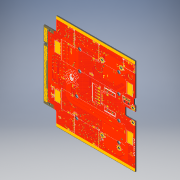
# Autodesk Inventor part: EPS_PCB
Saved by Autodesk Inventor 2018 (Build 220112000, 112)
## iProperties
Created: 2018-01-15
Part Number: EPS_PCB
Material: Epoxy Resin
Document SubType Name: Modeling
Designer: Bradley
Density: 1.14 g/cm^3
Appearance: Smooth - Dark Gray
Author: Bradley
Revision Number: 3
Autodesk Inventor part; units mm, degrees
ref_plane "YZ Plane" through (0, 0, 0) normal (1, 0, 0) x (0, 1, 0)
ref_plane "XZ Plane" through (0, 0, 0) normal (0, 1, 0) x (-1, 0, 0)
ref_plane "XY Plane" through (0, 0, 0) normal (0, 0, 1) x (1, 0, 0)
sketch "Sketch1" plane through (0, 0, 0) normal (0, 0, 1) x (1, 0, 0)
  line L0 (0, 33.8) -> (12.5, 33.8)
  line L1 (12.5, 33.8) -> (12.5, 47.9)
  line L2 (12.5, 47.9) -> (91.4, 47.9)
  line L3 (91.4, 47.9) -> (91.4, -47.9)
  line L4 (91.4, -47.9) -> (12.5, -47.9)
  line L5 (12.5, -47.9) -> (12.5, -33.8)
  line L6 (12.5, -33.8) -> (0, -33.8)
  line L7 (0, -33.8) -> (0, 33.8)
  line L8 (-4.5, 48) -> (91.5, 48) construction
  line L9 (91.5, 48) -> (91.5, -48) construction
  line L10 (91.5, -48) -> (-4.5, -48) construction
  line L11 (-4.5, -48) -> (-4.5, 48) construction
  line L12 (-4.4, 47.9) -> (-3.4, 47.9) construction
  line L13 (-3.4, 47.9) -> (-3.4, -47.9) construction
  line L14 (-3.4, -47.9) -> (-4.4, -47.9) construction
  line L15 (-4.4, -47.9) -> (-4.4, 47.9) construction
  point P0 (0, 0)
  point P1 (0, 0)
  point P2 (-4.5, 0)
  dimension "d0" = 67.6
  dimension "d1" = 95.8
  dimension "d2" = 91.4
  dimension "d3" = 12.5
  dimension "d20" = 96
  dimension "d21" = 96
  dimension "d22" = 0.1
  dimension "d23" = 0.1
  dimension "d24" = 1
  dimension "d25" = 0.1
  dimension "d26" = 3.4
  constraints: 32 end point, 8 perpendicular, 4 parallel, 3 collinear, 3 horizontal, 2 midpoint, 2 point on line, 1 coincident, 1 horizontal alignment
  measures "d0" distance of L6.end L0.start
  measures "d1" distance of L2.end L3.end
  measures "d2" distance between parallel lines of L7 L3
  measures "d3" distance of L0.start L0.end
  measures "d20" distance of L8.start L8.end
  measures "d21" distance of L10.end L8.start
  measures "d22" distance between parallel lines of L2 L8
  measures "d23" distance between parallel lines of L9 L3
  measures "d24" distance between parallel lines of L15 L13
  measures "d25" distance between parallel lines of L15 L11
  measures "d26" distance between parallel lines of L7 L13
extrude "Extrusion1" add sketch "Sketch1" along normal mid plane 1
sketch "Sketch3" plane through (0, 0, 0.5) normal (0, 0, 1) x (1, 0, 0)
  circle A0 centre (6, 31.8) radius 0.9
  circle A1 centre (6, -31.8) radius 0.9
  point P0 (0, 0)
  dimension "d9" = 1.8
  dimension "d10" = 6
  dimension "d11" = 31.8
  dimension "d12" = 31.8
  constraints: 2 centre point, 1 equal radius, 1 vertical alignment
  measures "d9" diameter of A0
  measures "d10" horizontal distance of point (0, 0) A0.centre
  measures "d11" vertical distance of point (0, 0) A0.centre
  measures "d12" vertical distance of A1.centre point (0, 0)
extrude "Extrusion3" cut sketch "Sketch3" against normal through all
sketch "Sketch4" plane through (0, 0, 0.5) normal (0, 0, 1) x (1, 0, 0)
  circle A0 centre (6, 31.8) radius 0.9 projected
  circle A1 centre (6, -31.8) radius 0.9 projected
  line L0 (91.4, -47.9) -> (91.4, 47.9) projected
  line L1 (12.5, 47.9) -> (12.5, 33.8) projected
  line L2 (12.5, 33.8) -> (0, 33.8) projected
  line L3 (0, 33.8) -> (0, -33.8) projected
  line L4 (0, -33.8) -> (12.5, -33.8) projected
  line L5 (12.5, -33.8) -> (12.5, -47.9) projected
  line L6 (0, 18.95) -> (3.5, 18.95)
  arc A2 (3.5, 17.95) -> (3.5, 18.95) centre (3.5, 18.45) ccw
  line L7 (3.5, 17.95) -> (0, 17.95)
  line L8 (12.5, -47.9) -> (91.4, -47.9) projected
  line L9 (91.4, 47.9) -> (12.5, 47.9) projected
  point P0 (0, 0)
  dimension "d15" = 17.95
  dimension "d16" = 3.5
  dimension "d17" = 1
  constraints: 4 end point, 2 point on circle, 2 point on line, 2 tangent, 1 centre point, 1 horizontal, 1 perpendicular
  measures "d15" distance from line of point (0, 0) L7
  measures "d16" distance from line of A2.centre L3
  measures "d17" distance between parallel lines of L7 L6
extrude "Extrusion4" cut sketch "Sketch4" against normal through all contours L3 L6 A2 L7
sketch "Sketch5" plane through (0, 0, 0.5) normal (0, 0, 1) x (1, 0, 0)
  line L0 (89.1, 6.3) -> (89.1, -6.3) construction
  line L1 (91.4, -47.9) -> (91.4, 47.9) projected
  line L2 (0, 17.95) -> (0, -33.8) projected
  point P0 (0, 0)
  point P1 (89.1, 0)
  point P2 (91.4, 0)
  point P3 (91.4, -45.4)
  point P4 (91.4, 45.4)
  dimension "d29" = 12.6
  dimension "d69" = 89.1
  constraints: 2 coincident, 2 end point, 2 midpoint, 1 horizontal alignment, 1 vertical
  measures "d29" distance of L0.start L0.end
  measures "d69" distance between parallel lines of L0 L2
hole "Hole1" at (89.1, 6.3, 0.5) at (89.1, -6.3, 0.5) direction (0, 0, -1) diameter 2.2 end through all clearance for "Socket Head Cap Screw" size "M2" standard "Ansi Metric M Profile"
sketch "Sketch6" plane through (0, 0, 0.5) normal (0, 0, 1) x (1, 0, 0)
  circle A0 centre (89.1, 6.3) radius 1.1 projected
  circle A1 centre (89.1, -6.3) radius 1.1 projected
  line L0 (0, 18.95) -> (3.5, 18.95) projected
  arc A2 (3.5, 17.95) -> (3.5, 18.95) centre (3.5, 18.45) ccw projected
  line L1 (3.5, 17.95) -> (0, 17.95) projected
  line L2 (0, 17.95) -> (0, -33.8) projected
  line L3 (0, -33.8) -> (12.5, -33.8) projected
  line L4 (12.5, -33.8) -> (12.5, -47.9) projected
  line L5 (91.4, -47.9) -> (91.4, 47.9) projected
  line L6 (12.5, 47.9) -> (12.5, 33.8) projected
  line L7 (12.5, 33.8) -> (0, 33.8) projected
  line L8 (0, 33.8) -> (0, 18.95) projected
  circle A3 centre (6, -31.8) radius 0.9 projected
  circle A4 centre (6, 31.8) radius 0.9 projected
  line L9 (91.4, 45.4) -> (91.4, -45.4) projected
  line L10 (91.4, 4) -> (82.4, 4)
  arc A5 (82.4, 4) -> (81.4, 3) centre (82.4, 3) ccw
  line L11 (81.4, 3) -> (81.4, -3)
  arc A6 (81.4, -3) -> (82.4, -4) centre (82.4, -3) ccw
  line L12 (82.4, -4) -> (91.4, -4)
  circle A7 centre (90.7, 13.2) radius 0.7 construction
  circle A8 centre (90.7, 11.8) radius 0.7 construction
  line L13 (91.4, 15.5) -> (90.9, 15.5)
  arc A9 (90.9, 15.5) -> (89.9, 14.5) centre (90.9, 14.5) ccw
  line L14 (89.9, 14.5) -> (89.9, 10.5)
  arc A10 (89.9, 10.5) -> (90.9, 9.5) centre (90.9, 10.5) ccw
  line L15 (90.9, 9.5) -> (91.4, 9.5)
  line L16 (91.4, -45.4) -> (91.4, 45.4) construction
  line L17 (89.9, 12.5) -> (91.4, 12.5) construction
  line L18 (12.5, -47.9) -> (91.4, -47.9) projected
  line L19 (91.4, 47.9) -> (12.5, 47.9) projected
  point P0 (0, 0)
  point P1 (81.4, 0)
  dimension "d37" = 1
  dimension "d38" = 8
  dimension "d39" = 1.2
  dimension "d40" = 10
  dimension "d65" = 1.4
  dimension "d66" = 1.5
  dimension "d67" = 6
  dimension "d68" = 12.5
  dimension "d70" = 9.5
  dimension "d71" = 15.5
  constraints: 14 end point, 12 tangent, 8 point on circle, 7 perpendicular, 6 centre point, 5 point on line, 3 equal radius, 2 midpoint, 1 horizontal alignment, 1 parallel
  measures "d37" radius of A5
  measures "d38" distance between parallel lines of L12 L10
  measures "d39" distance edge to line of A0 L10
  measures "d40" distance between parallel lines of L5 L11
  measures "d65" diameter of A7
  measures "d66" distance between parallel lines of L5 L14
  measures "d67" distance between parallel lines of L15 L13
  measures "d68" distance from line of point (0, 0) L17
  measures "d70" distance from line of L15 point (0, 0)
  measures "d71" distance from line of point (0, 0) L13
extrude "Extrusion5" cut sketch "Sketch6" against normal through all contours L5 L15 A10 L14 A9 L13 | L5 L12 A6 L11 A5 L10
sketch "Sketch7" plane through (0, 0, 0.5) normal (0, 0, 1) x (1, 0, 0)
  line L0 (80.65, 7.93) -> (84.65, 7.93) construction
  line L1 (91.4, 4) -> (91.4, 9.5) projected
  point P0 (0, 0)
  point P1 (91.4, 45.4)
  dimension "d43" = 7.93
  dimension "d44" = 6.75
  dimension "d45" = 4
  constraints: 2 coincident, 2 end point, 1 horizontal
  measures "d43" distance from line of point (0, 0) L0
  measures "d44" distance from line of L1 L0.end
  measures "d45" distance of L0.start L0.end
hole "Hole2" at (80.65, 7.93, 0.5) at (84.65, 7.93, 0.5) direction (0, 0, -1) diameter 1.7 end through all
fillet "Fillet1" radius 0.5 12 edges at (91.4, 4, 0) (91.4, -4, 0) (91.4, 9.5, 0) (91.4, 15.5, 0) (91.4, 47.9, 0) (12.5, 47.9, 0) (0, 33.8, 0) (0, 18.95, 0) (0, 17.95, 0) (0, -33.8, 0) (12.5, -47.9, 0) (91.4, -47.9, 0)
fillet "Fillet1" radius 1 2 edges at (12.5, 33.8, 0) (12.5, -33.8, 0)
sketch "Sketch8" plane through (0, 0, 0.5) normal (0, 0, 1) x (1, 0, 0)
  arc A0 (91.4, -4.5) -> (90.9, -4) centre (90.9, -4.5) ccw projected
  line L0 (90.9, -4) -> (82.4, -4) projected
  arc A1 (81.4, -3) -> (82.4, -4) centre (82.4, -3) ccw projected
  line L1 (81.4, -3) -> (81.4, 3) projected
  arc A2 (82.4, 4) -> (81.4, 3) centre (82.4, 3) ccw projected
  line L2 (82.4, 4) -> (90.9, 4) projected
  arc A3 (90.9, 4) -> (91.4, 4.5) centre (90.9, 4.5) ccw projected
  line L3 (91.4, 4.5) -> (91.4, 9) projected
  line L4 (12.5, 47.4) -> (12.5, 34.8) projected
  arc A4 (11.5, 33.8) -> (12.5, 34.8) centre (11.5, 34.8) ccw projected
  line L5 (11.5, 33.8) -> (0.5, 33.8) projected
  line L6 (0, 17.45) -> (0, -33.3) projected
  line L7 (0.5, 18.95) -> (3.5, 18.95) projected
  arc A5 (3.5, 17.95) -> (3.5, 18.95) centre (3.5, 18.45) ccw projected
  line L8 (3.5, 17.95) -> (0.5, 17.95) projected
  line L9 (0, 33.3) -> (0, 19.45) projected
  line L10 (0.5, -33.8) -> (11.5, -33.8) projected
  arc A6 (12.5, -34.8) -> (11.5, -33.8) centre (11.5, -34.8) ccw projected
  line L11 (12.5, -34.8) -> (12.5, -47.4) projected
  line L12 (91.4, 16) -> (91.4, 47.4) projected
  circle A7 centre (80.65, 7.93) radius 0.85 projected
  circle A8 centre (84.65, 7.93) radius 0.85 projected
  circle A9 centre (6, 31.8) radius 0.9 projected
  circle A10 centre (6, -31.8) radius 0.9 projected
  circle A11 centre (89.1, -6.3) radius 1.1 projected
  circle A12 centre (89.1, 6.3) radius 1.1 projected
  line L13 (75, 30.5) -> (75, 11.5) construction
  line L14 (33, -11.5) -> (33, -30.5) construction
  line L15 (75, -11.5) -> (75, -30.5) construction
  line L16 (0, 0) -> (81.4, 0) construction
  arc A13 (89.9, 10.5) -> (90.9, 9.5) centre (90.9, 10.5) ccw projected
  line L17 (89.9, 10.5) -> (89.9, 14.5) projected
  arc A14 (90.9, 15.5) -> (89.9, 14.5) centre (90.9, 14.5) ccw projected
  line L18 (91.4, -47.4) -> (91.4, -4.5) projected
  arc A15 (90.9, 15.5) -> (91.4, 16) centre (90.9, 16) ccw projected
  arc A16 (91.4, 9) -> (90.9, 9.5) centre (90.9, 9) ccw projected
  arc A17 (90.9, -47.9) -> (91.4, -47.4) centre (90.9, -47.4) ccw projected
  arc A18 (91.4, 47.4) -> (90.9, 47.9) centre (90.9, 47.4) ccw projected
  line L19 (90.9, 47.9) -> (13, 47.9) projected
  arc A19 (13, 47.9) -> (12.5, 47.4) centre (13, 47.4) ccw projected
  arc A20 (0.5, 33.8) -> (0, 33.3) centre (0.5, 33.3) ccw projected
  arc A21 (0, 19.45) -> (0.5, 18.95) centre (0.5, 19.45) ccw projected
  arc A22 (0.5, 17.95) -> (0, 17.45) centre (0.5, 17.45) ccw projected
  arc A23 (0, -33.3) -> (0.5, -33.8) centre (0.5, -33.3) ccw projected
  arc A24 (12.5, -47.4) -> (13, -47.9) centre (13, -47.4) ccw projected
  line L20 (13, -47.9) -> (90.9, -47.9) projected
  line L21 (36, 30.5) -> (36, 11.5) construction
  point P0 (75, 21)
  point P1 (75, -21)
  point P2 (33, -21)
  dimension "d54" = 21
  dimension "d55" = 33
  dimension "d56" = 75
  dimension "d57" = 19
  dimension "d73" = 36
  constraints: 10 end point, 6 coincident, 4 midpoint, 4 vertical, 3 horizontal alignment, 2 symmetric about line, 1 parallel
  measures "d54" vertical distance of point (33, -21) L16.start
  measures "d55" distance between parallel lines of L14 L9
  measures "d56" distance between parallel lines of L15 L9
  measures "d57" distance of L14.start L14.end
  measures "d73" distance between parallel lines of L9 L21
hole "Hole3" at (36, 30.5, 0.5) at (36, 11.5, 0.5) at (75, 11.5, 0.5) at (75, 30.5, 0.5) at (75, -11.5, 0.5) at (75, -30.5, 0.5) at (33, -30.5, 0.5) at (33, -11.5, 0.5) direction (0, 0, -1) diameter 3 end through all
sketch "Sketch10" plane through (0, 0, 0.5) normal (0, 0, 1) x (1, 0, 0)
  line L0 (0, 33.3) -> (0, 19.45) projected
  point P0 (0, 0)
  point P1 (58.3, 32.5)
  point P2 (77.3, 35)
  point P3 (58.4, -32.5)
  point P4 (75.1, -35)
  dimension "d74" = 58.3
  dimension "d75" = 32.5
  dimension "d76" = 35
  dimension "d77" = 77.3
  dimension "d78" = 75.1
  dimension "d79" = 35
  dimension "d80" = 32.5
  dimension "d81" = 58.4
  measures "d74" distance from line of point (58.3, 32.5) L0
  measures "d75" vertical distance of point (0, 0) point (58.3, 32.5)
  measures "d76" vertical distance of point (0, 0) point (77.3, 35)
  measures "d77" horizontal distance of point (77.3, 35) point (0, 0)
  measures "d78" horizontal distance of point (75.1, -35) point (0, 0)
  measures "d79" vertical distance of point (0, 0) point (75.1, -35)
  measures "d80" vertical distance of point (0, 0) point (58.4, -32.5)
  measures "d81" horizontal distance of point (58.4, -32.5) point (0, 0)
hole "Hole4" at (58.3, 32.5, 0.5) at (77.3, 35, 0.5) at (58.4, -32.5, 0.5) at (75.1, -35, 0.5) direction (0, 0, -1) diameter 2.2 end through all
sketch "Sketch11" plane through (0, 0, 0.5) normal (0, 0, 1) x (1, 0, 0)
  line L0 (0, 47.8798) -> (91.4, 47.8798) construction
  line L1 (91.4, 47.8798) -> (91.4, -47.8798) construction
  line L2 (91.4, -47.8798) -> (0, -47.8798) construction
  line L3 (0, -47.8798) -> (0, 47.8798) construction
  circle A0 centre (58.4, -32.5) radius 1.1 projected
  circle A1 centre (58.3, 32.5) radius 1.1 projected
  circle A2 centre (77.3, 35) radius 1.1 projected
  circle A3 centre (75.1, -35) radius 1.1 projected
  circle A4 centre (33, -30.5) radius 1.5 projected
  circle A5 centre (75, -11.5) radius 1.5 projected
  circle A6 centre (75, 11.5) radius 1.5 projected
  circle A7 centre (36, 30.5) radius 1.5 projected
  circle A8 centre (36, 11.5) radius 1.5 projected
  circle A9 centre (75, 30.5) radius 1.5 projected
  circle A10 centre (75, -30.5) radius 1.5 projected
  circle A11 centre (33, -11.5) radius 1.5 projected
  arc A12 (90.9, -47.9) -> (91.4, -47.4) centre (90.9, -47.4) ccw projected
  line L4 (91.4, -47.4) -> (91.4, -4.5) projected
  arc A13 (91.4, -4.5) -> (90.9, -4) centre (90.9, -4.5) ccw projected
  line L5 (90.9, -4) -> (82.4, -4) projected
  arc A14 (81.4, -3) -> (82.4, -4) centre (82.4, -3) ccw projected
  line L6 (81.4, -3) -> (81.4, 3) projected
  arc A15 (82.4, 4) -> (81.4, 3) centre (82.4, 3) ccw projected
  line L7 (82.4, 4) -> (90.9, 4) projected
  arc A16 (90.9, 4) -> (91.4, 4.5) centre (90.9, 4.5) ccw projected
  line L8 (91.4, 4.5) -> (91.4, 9) projected
  arc A17 (91.4, 9) -> (90.9, 9.5) centre (90.9, 9) ccw projected
  arc A18 (89.9, 10.5) -> (90.9, 9.5) centre (90.9, 10.5) ccw projected
  line L9 (89.9, 10.5) -> (89.9, 14.5) projected
  arc A19 (90.9, 15.5) -> (89.9, 14.5) centre (90.9, 14.5) ccw projected
  arc A20 (90.9, 15.5) -> (91.4, 16) centre (90.9, 16) ccw projected
  line L10 (91.4, 16) -> (91.4, 47.4) projected
  arc A21 (91.4, 47.4) -> (90.9, 47.9) centre (90.9, 47.4) ccw projected
  line L11 (90.9, 47.9) -> (13, 47.9) projected
  arc A22 (13, 47.9) -> (12.5, 47.4) centre (13, 47.4) ccw projected
  line L12 (12.5, 47.4) -> (12.5, 34.8) projected
  arc A23 (11.5, 33.8) -> (12.5, 34.8) centre (11.5, 34.8) ccw projected
  line L13 (11.5, 33.8) -> (0.5, 33.8) projected
  arc A24 (0.5, 33.8) -> (0, 33.3) centre (0.5, 33.3) ccw projected
  line L14 (0, 33.3) -> (0, 19.45) projected
  arc A25 (0, 19.45) -> (0.5, 18.95) centre (0.5, 19.45) ccw projected
  line L15 (0.5, 18.95) -> (3.5, 18.95) projected
  arc A26 (3.5, 17.95) -> (3.5, 18.95) centre (3.5, 18.45) ccw projected
  line L16 (3.5, 17.95) -> (0.5, 17.95) projected
  arc A27 (0.5, 17.95) -> (0, 17.45) centre (0.5, 17.45) ccw projected
  line L17 (0, 17.45) -> (0, -33.3) projected
  arc A28 (0, -33.3) -> (0.5, -33.8) centre (0.5, -33.3) ccw projected
  line L18 (0.5, -33.8) -> (11.5, -33.8) projected
  arc A29 (12.5, -34.8) -> (11.5, -33.8) centre (11.5, -34.8) ccw projected
  line L19 (12.5, -34.8) -> (12.5, -47.4) projected
  arc A30 (12.5, -47.4) -> (13, -47.9) centre (13, -47.4) ccw projected
  line L20 (13, -47.9) -> (90.9, -47.9) projected
  circle A31 centre (89.1, 6.3) radius 1.1 projected
  circle A32 centre (89.1, -6.3) radius 1.1 projected
  circle A33 centre (6, -31.8) radius 0.9 projected
  circle A34 centre (6, 31.8) radius 0.9 projected
  circle A35 centre (84.65, 7.93) radius 0.85 projected
  circle A36 centre (80.65, 7.93) radius 0.85 projected
  line L21 (0, 17.45) -> (0, -33.3) projected
  line L22 (91.4, 16) -> (91.4, 47.4) projected
  point P0 (0, 0)
  constraints: 2 collinear, 1 midpoint, 2 other
decal "Decal1"
sketch "Sketch12" plane through (0, 0, -0.5) normal (0, 0, -1) x (-1, 0, 0)
  circle A0 centre (-58.4, -32.5) radius 1.1 projected
  circle A1 centre (-58.3, 32.5) radius 1.1 projected
  circle A2 centre (-77.3, 35) radius 1.1 projected
  circle A3 centre (-75.1, -35) radius 1.1 projected
  circle A4 centre (-33, -30.5) radius 1.5 projected
  circle A5 centre (-75, -11.5) radius 1.5 projected
  circle A6 centre (-75, 11.5) radius 1.5 projected
  circle A7 centre (-36, 30.5) radius 1.5 projected
  circle A8 centre (-36, 11.5) radius 1.5 projected
  circle A9 centre (-75, 30.5) radius 1.5 projected
  circle A10 centre (-75, -30.5) radius 1.5 projected
  circle A11 centre (-33, -11.5) radius 1.5 projected
  circle A12 centre (-6, -31.8) radius 0.9 projected
  circle A13 centre (-6, 31.8) radius 0.9 projected
  circle A14 centre (-89.1, -6.3) radius 1.1 projected
  circle A15 centre (-89.1, 6.3) radius 1.1 projected
  circle A16 centre (-84.65, 7.93) radius 0.85 projected
  circle A17 centre (-80.65, 7.93) radius 0.85 projected
  arc A18 (-91.4, -47.4) -> (-90.9, -47.9) centre (-90.9, -47.4) ccw projected
  line L0 (-90.9, -47.9) -> (-13, -47.9) projected
  arc A19 (-13, -47.9) -> (-12.5, -47.4) centre (-13, -47.4) ccw projected
  line L1 (-12.5, -47.4) -> (-12.5, -34.8) projected
  arc A20 (-11.5, -33.8) -> (-12.5, -34.8) centre (-11.5, -34.8) ccw projected
  line L2 (-11.5, -33.8) -> (-0.5, -33.8) projected
  arc A21 (-0.5, -33.8) -> (0, -33.3) centre (-0.5, -33.3) ccw projected
  line L3 (0, -33.3) -> (0, 17.45) projected
  arc A22 (0, 17.45) -> (-0.5, 17.95) centre (-0.5, 17.45) ccw projected
  line L4 (-0.5, 17.95) -> (-3.5, 17.95) projected
  arc A23 (-3.5, 18.95) -> (-3.5, 17.95) centre (-3.5, 18.45) ccw projected
  line L5 (-3.5, 18.95) -> (-0.5, 18.95) projected
  arc A24 (-0.5, 18.95) -> (0, 19.45) centre (-0.5, 19.45) ccw projected
  line L6 (0, 19.45) -> (0, 33.3) projected
  arc A25 (0, 33.3) -> (-0.5, 33.8) centre (-0.5, 33.3) ccw projected
  line L7 (-0.5, 33.8) -> (-11.5, 33.8) projected
  arc A26 (-12.5, 34.8) -> (-11.5, 33.8) centre (-11.5, 34.8) ccw projected
  line L8 (-12.5, 34.8) -> (-12.5, 47.4) projected
  arc A27 (-12.5, 47.4) -> (-13, 47.9) centre (-13, 47.4) ccw projected
  line L9 (-13, 47.9) -> (-90.9, 47.9) projected
  arc A28 (-90.9, 47.9) -> (-91.4, 47.4) centre (-90.9, 47.4) ccw projected
  line L10 (-91.4, 47.4) -> (-91.4, 16) projected
  arc A29 (-91.4, 16) -> (-90.9, 15.5) centre (-90.9, 16) ccw projected
  arc A30 (-89.9, 14.5) -> (-90.9, 15.5) centre (-90.9, 14.5) ccw projected
  line L11 (-89.9, 14.5) -> (-89.9, 10.5) projected
  arc A31 (-90.9, 9.5) -> (-89.9, 10.5) centre (-90.9, 10.5) ccw projected
  arc A32 (-90.9, 9.5) -> (-91.4, 9) centre (-90.9, 9) ccw projected
  line L12 (-91.4, 9) -> (-91.4, 4.5) projected
  arc A33 (-91.4, 4.5) -> (-90.9, 4) centre (-90.9, 4.5) ccw projected
  line L13 (-90.9, 4) -> (-82.4, 4) projected
  arc A34 (-81.4, 3) -> (-82.4, 4) centre (-82.4, 3) ccw projected
  line L14 (-81.4, 3) -> (-81.4, -3) projected
  arc A35 (-82.4, -4) -> (-81.4, -3) centre (-82.4, -3) ccw projected
  line L15 (-82.4, -4) -> (-90.9, -4) projected
  arc A36 (-90.9, -4) -> (-91.4, -4.5) centre (-90.9, -4.5) ccw projected
  line L16 (-91.4, -4.5) -> (-91.4, -47.4) projected
  line L17 (0, -33.3) -> (0, 17.45) projected
  line L18 (-91.4, 47.8917) -> (0, 47.8917) construction
  line L19 (0, 47.8917) -> (0, -47.8917) construction
  line L20 (0, -47.8917) -> (-91.4, -47.8917) construction
  line L21 (-91.4, -47.8917) -> (-91.4, 47.8917) construction
  line L22 (-91.4, 47.4) -> (-91.4, 16) projected
  point P0 (0, 0)
  constraints: 2 collinear, 1 midpoint, 2 other
decal "Decal2"
sketch "Sketch13" plane through (0, 0, 0.5) normal (0, 0, 1) x (1, 0, 0)
  point P0 (0, 0)
  point P1 (89.96, 41.605)
  point P2 (61.8, 38.5)
  point P3 (62.4, 38.5)
  point P4 (62.4, 39.1)
  point P5 (63, 39.1)
  point P6 (63, 39.7)
  point P7 (40.8, 35.695)
  point P8 (61.1, 39.8)
  point P9 (60.5, 39.8)
  point P10 (60.5, 39.2)
  point P11 (59.9, 39.2)
  point P12 (59.9, 38.6)
  point P13 (34.6, 34.5)
  point P14 (33.21, -3.955)
  point P15 (35.14, -4.665)
  point P16 (38, -33.2)
  point P17 (42.6, -39.6)
  point P18 (40.095, -41.49)
  point P19 (54.71, -30.72)
  point P20 (50, -39.6)
  point P21 (47.5, -41.7)
  point P22 (29.8, 43.6)
  point P23 (51, 41.7)
  point P24 (40.6, 40.96)
  point P25 (43.1, 43.1)
  point P26 (58.4, -6.46)
  point P27 (76.84, -5.14)
  point P28 (77.5, 5.4)
  point P29 (55.26, -42.83)
  point P30 (27.48, -21.06)
  point P31 (36.425, -25.76)
  point P32 (88.9, 21.15)
  point P33 (89.45, 20.8)
  point P34 (88.9, 20.45)
  point P35 (89.45, 20.1)
  point P36 (88.9, 19.75)
  point P37 (89.45, 19.4)
  point P38 (88.9, 19.05)
  point P39 (79.82, -3.995)
  point P40 (85.12, 31.545)
  point P41 (52.8, 22)
  point P42 (51.16, 44.12)
  point P43 (36.315, 43.16)
  point P44 (34, 40.7)
  point P45 (29.26, -22.34)
  point P46 (56.36, -42.83)
  point P47 (86.1, -15.5)
  point P48 (86.8, -15.5)
  point P49 (87.5, -15.5)
  point P50 (88.2, -15.5)
  point P51 (88.9, -15.7)
  point P52 (89, -16.4)
  point P53 (89, -17.1)
  point P54 (89, -17.8)
  point P55 (89, -18.5)
  point P56 (36.38, -26.57)
  point P57 (78.1, -7)
  point P58 (79.355, -3.255)
  point P59 (51.1, 42.9)
  point P60 (10.2, -23.5)
  point P61 (7.6, -20.8)
  point P62 (10.4, -20.8)
  point P63 (11, -23.5)
  point P64 (10.2, -16.8)
  point P65 (7.6, -14.1)
  point P66 (11, -16.8)
  point P67 (10.85, -14.23)
  point P68 (16.5, -14.5)
  point P69 (16.5, -15.3)
  point P70 (17.1, -15.7)
  point P71 (17.1, -14.9)
  point P72 (17.1, -14.1)
  point P73 (26.79, -20.74)
  point P74 (53.3, -24.9)
  point P75 (65.155, 10.12)
  point P76 (52, 22.1)
  point P77 (20, 6.69)
  point P78 (20, 3.69)
  point P79 (20, 0.69)
  point P80 (24.54, 7.29)
  point P81 (24.1, 5.25)
  point P82 (24.1, 2.15)
  point P83 (24.125, -0.96)
  point P84 (78.3, -37.4)
  point P85 (81.2, -17.1)
  point P86 (81.2, -17.9)
  point P87 (81.2, -18.7)
  point P88 (81.2, -19.5)
  point P89 (80.6, -19.1)
  point P90 (80.6, -18.3)
  point P91 (80.6, -17.5)
  point P92 (79.5, -38.9)
  point P93 (60.7, -41.8)
  point P94 (54.9, -25.4)
  point P95 (49.9, -17.2)
  point P96 (78, -17)
  point P97 (77.2, -17)
  point P98 (75.3, 8)
  point P99 (75.7, 7.5)
  point P100 (74.9, 7.5)
  point P101 (86.23, 30.36)
  point P102 (87, 30.2)
  point P103 (16.5, 5.53)
  point P104 (16.5, 2.53)
  point P105 (16.5, -0.47)
  point P106 (21.1, 6.97)
  point P107 (21.1, 3.97)
  point P108 (21.1, 0.97)
  point P109 (21.1, -2.03)
  point P110 (17.6, -2.4)
  point P111 (18.4, -2.4)
  point P112 (19.2, -2.4)
  point P113 (20, -2.4)
  point P114 (20.4, -3.1)
  point P115 (19.6, -3.1)
  point P116 (18.8, -3.1)
  point P117 (18, -3.1)
  point P118 (28.5, -3.2)
  point P119 (28.5, -4)
  point P120 (28.5, -4.8)
  point P121 (28.5, -5.6)
  point P122 (29.1, -5.2)
  point P123 (29.1, -4.4)
  point P124 (29.1, -3.6)
  point P125 (27.6, 22.4)
  point P126 (27.6, 23)
  point P127 (27.6, 23.7)
  point P128 (27.6, 24.3)
  point P129 (27.05, 24)
  point P130 (27.1, 23.35)
  point P131 (28.5, -11.42)
  point P132 (32.13, -21.7)
  point P133 (21.2, -42.1)
  point P134 (29.295, -43.15)
  point P135 (34.66, -26.63)
  point P136 (54.85, -20.36)
  point P137 (56.64, -20.36)
  point P138 (73, 41.8)
  point P139 (84.36, 31.55)
  point P140 (53.67, 21.255)
  point P141 (58.1, 22.8)
  point P142 (19.26, -22.78)
  point P143 (43.945, -10.34)
  point P144 (79.28, 4.89)
  point P145 (79.375, 14.54)
  point P146 (83.96, 26.46)
  point P147 (43.4, -40.4)
  point P148 (52.1, -33.5)
  point P149 (40.1, -40.6)
  point P150 (49.4, -33.9)
  point P151 (50.7, -40.5)
  point P152 (52.6, -38)
  point P153 (47.64, -39.63)
  point P154 (51.6, -36.4)
  point P155 (35.23, 40.2)
  point P156 (35.395, 38.8)
  point P157 (37.02, 41.69)
  point P158 (36.155, 38.8)
  point P159 (40.545, 42.945)
  point P160 (37.685, 38.8)
  point P161 (43.645, 41.71)
  point P162 (40.18, 38.76)
  point P163 (60.01, -1.17)
  point P164 (77, -3.8)
  point P165 (64.23, -0.73)
  point P166 (59.32, -1.49)
  point P167 (77.56, -5.495)
  point P168 (64.255, -1.49)
  point P169 (28.24, -21.06)
  point P170 (53.1, -25.7)
  point P171 (26.13, -20.36)
  point P172 (54.1, -24.7)
  point P173 (15.8, 40.45)
  point P174 (22.3, 38.45)
  point P175 (15.3, -4.2)
  point P176 (17, -5.2)
  point P177 (13.71, -10.51)
  point P178 (29.895, -6.39)
  point P179 (25.4, 40.45)
  point P180 (31.6, 38)
  point P181 (31.12, 30.22)
  point P182 (28.48, -10.66)
  point P183 (19.6, -13.6)
  point P184 (28.9, -38.5)
  point P185 (27.58, -34.4)
  point P186 (47.6, -27.75)
  point P187 (44.2, -21.8)
  point P188 (37.24, -26.61)
  point P189 (35.26, -35.79)
  point P190 (57.925, 25.16)
  point P191 (51.6, 27.8)
  point P192 (51.6, 25.9)
  point P193 (47.97, 26.905)
  point P194 (43.625, 31.08)
  point P195 (71.1, -41.92)
  point P196 (55.7, -25.6)
  point P197 (20, 27.59)
  point P198 (21.9, 30.59)
  point P199 (20, 24.59)
  constraints: 629 other
hole "Hole5" at (89.96, 41.605, 0.5) at (61.8, 38.5, 0.5) at (62.4, 38.5, 0.5) at (62.4, 39.1, 0.5) at (63, 39.1, 0.5) at (63, 39.7, 0.5) at (40.8, 35.695, 0.5) at (61.1, 39.8, 0.5) at (60.5, 39.8, 0.5) at (60.5, 39.2, 0.5) at (59.9, 39.2, 0.5) at (59.9, 38.6, 0.5) at (34.6, 34.5, 0.5) at (33.21, -3.955, 0.5) at (35.14, -4.665, 0.5) at (38, -33.2, 0.5) at (42.6, -39.6, 0.5) at (40.095, -41.49, 0.5) at (54.71, -30.72, 0.5) at (50, -39.6, 0.5) at (47.5, -41.7, 0.5) at (29.8, 43.6, 0.5) at (51, 41.7, 0.5) at (40.6, 40.96, 0.5) at (43.1, 43.1, 0.5) at (58.4, -6.46, 0.5) at (76.84, -5.14, 0.5) at (77.5, 5.4, 0.5) at (55.26, -42.83, 0.5) at (27.48, -21.06, 0.5) at (36.425, -25.76, 0.5) at (88.9, 21.15, 0.5) at (89.45, 20.8, 0.5) at (88.9, 20.45, 0.5) at (89.45, 20.1, 0.5) at (88.9, 19.75, 0.5) at (89.45, 19.4, 0.5) at (88.9, 19.05, 0.5) at (79.82, -3.995, 0.5) at (85.12, 31.545, 0.5) at (52.8, 22, 0.5) at (51.16, 44.12, 0.5) at (36.315, 43.16, 0.5) at (34, 40.7, 0.5) at (29.26, -22.34, 0.5) at (56.36, -42.83, 0.5) at (86.1, -15.5, 0.5) at (86.8, -15.5, 0.5) at (87.5, -15.5, 0.5) at (88.2, -15.5, 0.5) direction (0, 0, -1) diameter 0.3 end through all and at (88.9, -15.7, 0.5) (89, -16.4, 0.5) (89, -17.1, 0.5) (89, -17.8, 0.5) (89, -18.5, 0.5) (36.38, -26.57, 0.5) (78.1, -7, 0.5) (79.355, -3.255, 0.5) (51.1, 42.9, 0.5) (10.2, -23.5, 0.5) (7.6, -20.8, 0.5) (10.4, -20.8, 0.5) (11, -23.5, 0.5) (10.2, -16.8, 0.5) (7.6, -14.1, 0.5) (11, -16.8, 0.5) (10.85, -14.23, 0.5) (16.5, -14.5, 0.5) (16.5, -15.3, 0.5) (17.1, -15.7, 0.5) (17.1, -14.9, 0.5) (17.1, -14.1, 0.5) (26.79, -20.74, 0.5) (53.3, -24.9, 0.5) (65.155, 10.12, 0.5) (52, 22.1, 0.5) (20, 6.69, 0.5) (20, 3.69, 0.5) (20, 0.69, 0.5) (24.54, 7.29, 0.5) (24.1, 5.25, 0.5) (24.1, 2.15, 0.5) (24.125, -0.96, 0.5) (78.3, -37.4, 0.5) (81.2, -17.1, 0.5) (81.2, -17.9, 0.5) (81.2, -18.7, 0.5) (81.2, -19.5, 0.5) (80.6, -19.1, 0.5) (80.6, -18.3, 0.5) (80.6, -17.5, 0.5) (79.5, -38.9, 0.5) (60.7, -41.8, 0.5) (54.9, -25.4, 0.5) (49.9, -17.2, 0.5) (78, -17, 0.5) (77.2, -17, 0.5) (75.3, 8, 0.5) (75.7, 7.5, 0.5) (74.9, 7.5, 0.5) (86.23, 30.36, 0.5) (87, 30.2, 0.5) (16.5, 5.53, 0.5) (16.5, 2.53, 0.5) (16.5, -0.47, 0.5) (21.1, 6.97, 0.5) (21.1, 3.97, 0.5) (21.1, 0.97, 0.5) (21.1, -2.03, 0.5) (17.6, -2.4, 0.5) (18.4, -2.4, 0.5) (19.2, -2.4, 0.5) (20, -2.4, 0.5) (20.4, -3.1, 0.5) (19.6, -3.1, 0.5) (18.8, -3.1, 0.5) (18, -3.1, 0.5) (28.5, -3.2, 0.5) (28.5, -4, 0.5) (28.5, -4.8, 0.5) (28.5, -5.6, 0.5) (29.1, -5.2, 0.5) (29.1, -4.4, 0.5) (29.1, -3.6, 0.5) (27.6, 22.4, 0.5) (27.6, 23, 0.5) (27.6, 23.7, 0.5) (27.6, 24.3, 0.5) (27.05, 24, 0.5) (27.1, 23.35, 0.5) (28.5, -11.42, 0.5) (32.13, -21.7, 0.5) (21.2, -42.1, 0.5) (29.295, -43.15, 0.5) (34.66, -26.63, 0.5) (54.85, -20.36, 0.5) (56.64, -20.36, 0.5) (73, 41.8, 0.5) (84.36, 31.55, 0.5) (53.67, 21.255, 0.5) (58.1, 22.8, 0.5) (19.26, -22.78, 0.5) (43.945, -10.34, 0.5) (79.28, 4.89, 0.5) (79.375, 14.54, 0.5) (83.96, 26.46, 0.5) (43.4, -40.4, 0.5) (52.1, -33.5, 0.5) (40.1, -40.6, 0.5) (49.4, -33.9, 0.5) (50.7, -40.5, 0.5) (52.6, -38, 0.5) (47.64, -39.63, 0.5) (51.6, -36.4, 0.5) (35.23, 40.2, 0.5) (35.395, 38.8, 0.5) (37.02, 41.69, 0.5) (36.155, 38.8, 0.5) (40.545, 42.945, 0.5) (37.685, 38.8, 0.5) (43.645, 41.71, 0.5) (40.18, 38.76, 0.5) (60.01, -1.17, 0.5) (77, -3.8, 0.5) (64.23, -0.73, 0.5) (59.32, -1.49, 0.5) (77.56, -5.495, 0.5) (64.255, -1.49, 0.5) (28.24, -21.06, 0.5) (53.1, -25.7, 0.5) (26.13, -20.36, 0.5) (54.1, -24.7, 0.5) (15.8, 40.45, 0.5) (22.3, 38.45, 0.5) (15.3, -4.2, 0.5) (17, -5.2, 0.5) (13.71, -10.51, 0.5) (29.895, -6.39, 0.5) (25.4, 40.45, 0.5) (31.6, 38, 0.5) (31.12, 30.22, 0.5) (28.48, -10.66, 0.5) (19.6, -13.6, 0.5) (28.9, -38.5, 0.5) (27.58, -34.4, 0.5) (47.6, -27.75, 0.5) (44.2, -21.8, 0.5) (37.24, -26.61, 0.5) (35.26, -35.79, 0.5) (57.925, 25.16, 0.5) (51.6, 27.8, 0.5) (51.6, 25.9, 0.5) (47.97, 26.905, 0.5) (43.625, 31.08, 0.5) (71.1, -41.92, 0.5) (55.7, -25.6, 0.5) (20, 27.59, 0.5) (21.9, 30.59, 0.5) (20, 24.59, 0.5) (20, 21.59, 0.5) (20.02, 18.59, 0.5) (20, 9.69, 0.5) (24.1, 20.15, 0.5) (24.1, 23.15, 0.5) (24.1, 26.15, 0.5) (24.4, 16.55, 0.5) (24.1, 11.25, 0.5) (24.4, 28.5, 0.5) (19.96, 12.37, 0.5) (21.9, 34.1, 0.5) (23.7, 34.2, 0.5) (41.3, -36.9, 0.5) (48.34, -33.38, 0.5) (48.1, -31.9, 0.5) (48.35, -29, 0.5) (65.4, -16, 0.5) (66.1, -16, 0.5) (66.9, -16, 0.5) (67.6, -16, 0.5) (41.435, -38.41, 0.5) (23.4, -43.5, 0.5) (36.84, -42.33, 0.5) (37.88, -29.865, 0.5) (46.6, -16.2, 0.5) (63.9, -14.4, 0.5) (55.4, 42.1, 0.5) (56.28, 38.63, 0.5) (64.7, 40.6, 0.5) (58.1, 22, 0.5) (16.5, 11.53, 0.5) (16.5, 8.53, 0.5) (16.5, 29.43, 0.5) (17, 26.43, 0.5) (17, 23.43, 0.5) (17, 20.43, 0.5) (17, 17.43, 0.5) (21.1, 27.87, 0.5) (21.1, 24.87, 0.5) (21.1, 21.87, 0.5) (21.1, 18.93, 0.5) (21.35, 15.3, 0.5) (21.1, 9.97, 0.5) (26.8, 26.1, 0.5) (27.6, 26.1, 0.5) (27.6, 25.3, 0.5) (26.8, 25.3, 0.5) (27.3, 26.7, 0.5) (38.3, -38.56, 0.5) (46.87, -33.38, 0.5) (22.645, -43.655, 0.5) (36.08, -42.33, 0.5) (45.8, -30.9, 0.5) (37.34, -29.33, 0.5) (69.4, 18.8, 0.5) (65.945, 14.36, 0.5) (65.845, 10.44, 0.5) (55.96, 20.465, 0.5) (57.4, 39.7, 0.5) (58.2, 38.9, 0.5) (64, 18.7, 0.5) (56.5, 21, 0.5) (3.5, 31.2, 0.5) (7.2, 28.5, 0.5) (3.5, 30, 0.5) (14.1, 34.79, 0.5) (3.5, 28.8, 0.5) (13.68, 28.04, 0.5) (21.36, 34.89, 0.5) (7.2, 25.5, 0.5) (3.5, 27.6, 0.5) (14.74, 36.17, 0.5) (11, 23.8, 0.5) (3.5, 26.4, 0.5) (22.5, 35.8, 0.5) (7.2, 22.5, 0.5) (3.5, 25.2, 0.5) (15.6, 37.4, 0.5) (10.55, 21.5, 0.5) (3.5, 24, 0.5) (22.48, 37.36, 0.5) (7, 19.8, 0.5) (3.5, 22.8, 0.5) (16.33, 34.7, 0.5) (3.5, 21.6, 0.5) (30.28, 16.29, 0.5) (30.96, 32.46, 0.5) (3.5, 20.4, 0.5) (29.64, 14.57, 0.5) (29.64, 31.49, 0.5) (3.5, 15.6, 0.5) (29.57, 13.81, 0.5) (25.28, 37.2, 0.5) (3.5, 14.4, 0.5) (15.56, 13.7, 0.5) (11.5, 12.96, 0.5) (28.69, 13.15, 0.5) (24.6, 35.8, 0.5) (3.5, 13.2, 0.5) (8.9, 11.4, 0.5) (12.05, -1.63, 0.5) (3.5, 12, 0.5) (12.42, 10.34, 0.5) (14.33, -2, 0.5) (3.5, 10.8, 0.5) (8.9, 8.4, 0.5) (8.86, -8.8, 0.5) (3.5, 9.6, 0.5) (12.4, 7.3, 0.5) (11.75, -10.5, 0.5) (3.5, 8.4, 0.5) (9.1, 5.4, 0.5) (10.04, -1.71, 0.5) (3.5, 7.2, 0.5) (12.4, 4.3, 0.5) (9.62, -9.85, 0.5) (3.5, 6, 0.5) (8.86, 2.53, 0.5) (9.05, -0.66, 0.5) (3.5, 4.8, 0.5) (7.2, 29.3, 0.5) (13.56, 34.25, 0.5) (14.51, 28.04, 0.5) (20.86, 34.31, 0.5) (7.2, 26.3, 0.5) (14.42, 35.48, 0.5) (11, 24.59, 0.5) (22.08, 35.16, 0.5) (7.2, 23.3, 0.5) (15.06, 36.86, 0.5) (10.85, 22.24, 0.5) (22.5, 36.57, 0.5) (7.9, 20.68, 0.5) (16.87, 34.16, 0.5) (30.98, 16.66, 0.5) (31.5, 31.88, 0.5) (30.4, 14.58, 0.5) (30.4, 31.49, 0.5) (30.095, 13.26, 0.5) (24.7, 36.6, 0.5) (16.24, 13.36, 0.5) (13.6, 12.9, 0.5) (24.9, 35.1, 0.5) (29.315, 12.715, 0.5) (9.6, 11.8, 0.5) (12.29, -0.9, 0.5) (39.1, -36, 0.5) (38.2, -37.6, 0.5) (34.1, 44, 0.5) (55.96, 37.94, 0.5) (13.26, 10.34, 0.5) (14.95, -1.56, 0.5) (9.52, 8.84, 0.5) (8.86, -9.56, 0.5) (13.2, 7.3, 0.5) (12.51, -10.55, 0.5) (9.72, 5.84, 0.5) (10.36, -2.4, 0.5) (13.2, 4.3, 0.5) (10.99, -10.55, 0.5) (9.56, 2.84, 0.5) (9.72, -1.02, 0.5) (84.4, 42.4, 0.5) (85.1, 42.4, 0.5) (84.36, 32.31, 0.5) (54.385, 20.995, 0.5) (84.76, 32.96, 0.5) (55.1, 20.735, 0.5) (61.01, 8.125, 0.5) (87.86, 30.28, 0.5) (67.72, -3.01, 0.5) (72.49, -4.865, 0.5) (64.39, 10.12, 0.5) (51.4, 23, 0.5) (43.87, -28.105, 0.5) (41.41, -23.115, 0.5) (42.66, -29.95, 0.5) (40.7, -23.4, 0.5) (41.1, -30.7, 0.5) (39, -24.4, 0.5) (72.5, -7.8, 0.5) (66.8, -7.2, 0.5) (42.005, -30.7, 0.5) (40, -24.4, 0.5) (73.04, -5.49, 0.5) (65.955, -7.28, 0.5) (13.7, 39.2, 0.5) (24.7, 38.2, 0.5) (47.46, -4.6, 0.5) (34.18, -0.94, 0.5) (34.18, 5.355, 0.5) (34.18, -3.11, 0.5) (34.4, 9.9, 0.5) (21.08, -11.93, 0.5) (19.38, -6.05, 0.5) (22.29, -38.9, 0.5) (20.3, -37, 0.5) (27.16, -33.765, 0.5) (18.8, -13.6, 0.5) (45, -37.5, 0.5) (37.745, -39.1, 0.5) (35.3, -39.1, 0.5) (38.5, -34.6, 0.5) (35.58, -34.6, 0.5) (43.035, -26.3, 0.5) (41.5, -27.1, 0.5) (57.35, -5.325, 0.5) (66.49, -0.11, 0.5) (55.14, 7.35, 0.5) (40.5, 13.1, 0.5) (47.6, 4.6, 0.5) (48.5, 36.6, 0.5) (51.6, 35.56, 0.5) (50.68, 32.15, 0.5) (48.66, 28.625, 0.5) (43.518, 37.283, 0.5) (58.13, 6.05, 0.5) (64.082, 0.182, 0.5) (20.2, -23.1, 0.5) (46.705, -8.49, 0.5) (17.9, -31.2, 0.5) (17.7, -28.75, 0.5) (55, 4.9, 0.5) (53.5, -8.585, 0.5) (52.06, -9.89, 0.5) (53.2, -1.2, 0.5) (53.09, -4.04, 0.5) (51.295, -9.89, 0.5) (18.7, -31.2, 0.5) (18.5, -29.55, 0.5) (50.3, -9.79, 0.5) (51.8, -3.7, 0.5) (22.1, 40.6, 0.5) (31.7, 40.6, 0.5) (31.8, 39, 0.5) (28.66, -35.25, 0.5) (17.85, -8.45, 0.5) (40.1, -35.15, 0.5) (45.7, -26.3, 0.5) (34.755, -7.73, 0.5) (45.3, 2.1, 0.5) (57.3, 29.2, 0.5) (52.625, 38.11, 0.5) (54.575, 30.57, 0.5) (22.1, 39.8, 0.5) (31.7, 39.8, 0.5) (28.98, -34.56, 0.5) (18.913, -8.243, 0.5) (40.1, -34.3, 0.5) (35.47, -7.99, 0.5) (44.95, -26.435, 0.5) (45.3, 2.9, 0.5) (57.9, 29.7, 0.5) (24.4, 41.9, 0.5) (53.82, 30.685, 0.5) (20.49, -24.5, 0.5) (50.305, -4.64, 0.5) (49.6, -8.5, 0.5) (21.58, -23.74, 0.5) (49.65, -4.25, 0.5) (48.8, -8.5, 0.5) (21.18, -24.82, 0.5) (53.325, -7.03, 0.5) (52.39, -4.36, 0.5) (20.89, -23.42, 0.5) (48.885, -3.48, 0.5) (45.395, -9.8, 0.5) (43.9, -41.9, 0.5) (46.3, -39.6, 0.5) (47.1, -40.4, 0.5) (52.6, -34.5, 0.5) (43.6, -41.2, 0.5) (51.6, -35.2, 0.5) (53.7, -39.6, 0.5) (51.3, -41.9, 0.5) (54.38, -40.5, 0.5) (55.6, -36, 0.5) (51.15, -41.12, 0.5) (55.6, -37.5, 0.5) (39.8, 43.1, 0.5) (36.795, 40.96, 0.5) (37.29, 42.405, 0.5) (36.92, 38.8, 0.5) (40.42, 41.7, 0.5) (38.45, 38.8, 0.5) (47.635, 41.37, 0.5) (43.775, 40.96, 0.5) (43.735, 42.54, 0.5) (38.635, 36.905, 0.5) (46.995, 40.96, 0.5) (39.905, 36.905, 0.5) (59.6, 7.915, 0.5) (85.06, 30.72, 0.5) (4.8, -27.3, 0.5) (5.17, -28.06, 0.5) (5.6, -28.91, 0.5) (6.2, -29.76, 0.5) (10.8, -32.625, 0.5) (15.6, -32.8, 0.5) (30.585, -6.07, 0.5) (31.98, 31.29, 0.5) (28.82, -12.115, 0.5) (30.025, -22.34, 0.5) (30.06, -28.32, 0.5) (48.22, -25.9, 0.5) (49.545, 27.36, 0.5) (43.09, 31.62, 0.5) (16.9, -21.2, 0.5) (16.9, -22, 0.5) (16.9, -22.8, 0.5) (17.5, -22.4, 0.5) (17.5, -21.6, 0.5) (28.25, -21.82, 0.5) (52.19, -25.965, 0.5) (61.26, 10.44, 0.5) (51.2, 24.1, 0.5) (22.4, -42.9, 0.5) (30.815, -43.15, 0.5) (85.38, 29.64, 0.5) (63.045, 9.48, 0.5) (32.205, 30.54, 0.5) (22.34, -38.11, 0.5) (17.535, -38.2, 0.5) (88.54, -43.43, 0.5) (90.2, -41.3, 0.5) (40.805, -43.47, 0.5) (35.39, -42.01, 0.5) (36.7, -27.26, 0.5) (30.785, -22.34, 0.5) (29.595, -13.44, 0.5) (50.83, -8.81, 0.5) (39, -8.5, 0.5) (31.7, -6.6, 0.5) (89.3, 44.4, 0.5) (63.605, 44.44, 0.5) (55.595, 29.605, 0.5) (52.545, -11.07, 0.5) (29.96, -27.565, 0.5) (21.6, -42.8, 0.5) (30.055, -43.15, 0.5) (62.02, 10.44, 0.5) (53.4, 37.99, 0.5) (90.8, -40.7, 0.5) (88.4, -42.5, 0.5) (58.6, -42.8, 0.5) (79.9, -42.8, 0.5) (79.3, 30.8, 0.5) (88.82, 31.305, 0.5) (90.5, 44.5, 0.5) (70.5, -3.945, 0.5) (59.085, -5.67, 0.5) (51.1, -4.6, 0.5) (43, -8.8, 0.5) (15.4, 41.9, 0.5) (48.21, -4.8, 0.5) (17.19, -8.07, 0.5) (25.5, -35.4, 0.5) (26.9, -26.9, 0.5) (44.995, -27.225, 0.5) (40.175, -31.34, 0.5) (28.98, -28.415, 0.5) (37.035, -9.1, 0.5) (43.19, -4.04, 0.5) (47.02, 3.44, 0.5) (52.3, 8.8, 0.5) (54.495, -2.85, 0.5) (55.7, 9.4, 0.5) (57.995, 24.4, 0.5) (49.305, 28.085, 0.5) (49.5, 32.1, 0.5) (36.09, 33.24, 0.5) (33.493, 29.9, 0.5) (33.293, 27.86, 0.5) (32.2, -9.05, 0.5) (32.8, -8.7, 0.5) (32.8, -9.4, 0.5) (86.1, -27.6, 0.5) (68.9, -20.8, 0.5) (69.4, -21.3, 0.5) (73.1, -21.3, 0.5) (73.6, -20.8, 0.5) (60.7, -20.7, 0.5) (61.4, -29.6, 0.5) (63.6, -29.6, 0.5) (63.6, -30.3, 0.5) (61.4, -30.3, 0.5) (59.9, -38.8, 0.5) (64.8, -41.6, 0.5) (68, -41.2, 0.5) (68.6, -40.8, 0.5) (68.6, -41.6, 0.5) (80.2, -37.7, 0.5) (58.8, -26, 0.5) (59.5, -40.7, 0.5) (82.715, -6.64, 0.5) (73.9, 0.2, 0.5) (74.38, -3.69, 0.5) (69.2, -0.2, 0.5) (37.6, 21, 0.5) (40.9, 16, 0.5) (79.3, 12.7, 0.5) (78.3, 40.2, 0.5) (79, 40.2, 0.5) (79.7, 40.2, 0.5) (80.4, 40.2, 0.5) (73, 36.3, 0.5) (73.7, 36.3, 0.5) (73.7, 34.5, 0.5) (73, 34.5, 0.5) (71.9, 28.6, 0.5) (71.9, 27.9, 0.5) (69.9, 27.9, 0.5) (69.9, 28.6, 0.5) (78.3, 29, 0.5) (59.5, 17.7, 0.5) (59.5, 18.4, 0.5) (59.5, 19.1, 0.5) (59.5, 19.8, 0.5) (60.1, 20.1, 0.5) (60.8, 20.1, 0.5) (63.8, 22.2, 0.5) (63.8, 21.5, 0.5) (63.8, 20.8, 0.5) (69.4, 16.4, 0.5) (88.18, 33.815, 0.5) (88.18, 33.195, 0.5) (88.18, 32.5, 0.5) (89.26, 42.305, 0.5) (89.96, 42.305, 0.5) (57.4, 21.4, 0.5)
sketch "Sketch14" plane through (0, 0, 0.5) normal (0, 0, 1) x (1, 0, 0)
  point P0 (0, 0)
  point P1 (90.7, -6.3)
  point P2 (89.1, -4.7)
  point P3 (87.969, -5.169)
  point P4 (87.5, -6.3)
  point P5 (87.969, -7.431)
  point P6 (89.1, -7.9)
  point P7 (90.231, -7.431)
  point P8 (90.231, -5.169)
  point P9 (90.7, 6.3)
  point P10 (90.231, 7.431)
  point P11 (89.1, 7.9)
  point P12 (90.231, 5.169)
  point P13 (87.969, 5.169)
  point P14 (56.7, 32.5)
  point P15 (57.169, 31.369)
  point P16 (58.3, 30.9)
  point P17 (59.431, 31.369)
  point P18 (59.9, 32.5)
  point P19 (59.431, 33.631)
  point P20 (58.3, 34.1)
  point P21 (57.169, 33.631)
  point P22 (87.5, 6.3)
  point P23 (75.7, 35)
  point P24 (76.169, 33.869)
  point P25 (77.3, 33.4)
  point P26 (78.431, 33.869)
  point P27 (78.9, 35)
  point P28 (78.431, 36.131)
  point P29 (77.3, 36.6)
  point P30 (76.169, 36.131)
  point P31 (87.969, 7.431)
  point P32 (76.7, -35)
  point P33 (76.231, -33.869)
  point P34 (75.1, -33.4)
  point P35 (22.41, 42.13)
  point P36 (73.5, -35)
  point P37 (73.969, -36.131)
  point P38 (75.1, -36.6)
  point P39 (76.231, -36.131)
  point P40 (89.1, 4.7)
  point P41 (60, -32.5)
  point P42 (73.969, -33.869)
  point P43 (58.4, -30.9)
  point P44 (57.269, -31.369)
  point P45 (56.8, -32.5)
  point P46 (57.269, -33.631)
  point P47 (58.4, -34.1)
  point P48 (59.531, -33.631)
  point P49 (59.531, -31.369)
  constraints: 49 other
hole "Hole6" at (90.7, -6.3, 0.5) at (89.1, -4.7, 0.5) at (87.969, -5.169, 0.5) at (87.5, -6.3, 0.5) at (87.969, -7.431, 0.5) at (89.1, -7.9, 0.5) at (90.231, -7.431, 0.5) at (90.231, -5.169, 0.5) at (90.7, 6.3, 0.5) at (90.231, 7.431, 0.5) at (89.1, 7.9, 0.5) at (90.231, 5.169, 0.5) at (87.969, 5.169, 0.5) at (56.7, 32.5, 0.5) at (57.169, 31.369, 0.5) at (58.3, 30.9, 0.5) at (59.431, 31.369, 0.5) at (59.9, 32.5, 0.5) at (59.431, 33.631, 0.5) at (58.3, 34.1, 0.5) at (57.169, 33.631, 0.5) at (87.5, 6.3, 0.5) at (75.7, 35, 0.5) at (76.169, 33.869, 0.5) at (77.3, 33.4, 0.5) at (78.431, 33.869, 0.5) at (78.9, 35, 0.5) at (78.431, 36.131, 0.5) at (77.3, 36.6, 0.5) at (76.169, 36.131, 0.5) at (87.969, 7.431, 0.5) at (76.7, -35, 0.5) at (76.231, -33.869, 0.5) at (75.1, -33.4, 0.5) at (22.41, 42.13, 0.5) at (73.5, -35, 0.5) at (73.969, -36.131, 0.5) at (75.1, -36.6, 0.5) at (76.231, -36.131, 0.5) at (89.1, 4.7, 0.5) at (60, -32.5, 0.5) at (73.969, -33.869, 0.5) at (58.4, -30.9, 0.5) at (57.269, -31.369, 0.5) at (56.8, -32.5, 0.5) at (57.269, -33.631, 0.5) at (58.4, -34.1, 0.5) at (59.531, -33.631, 0.5) at (59.531, -31.369, 0.5) direction (0, 0, -1) diameter 0.35 end through all
sketch "Sketch15" plane through (0, 0, 0.5) normal (0, 0, 1) x (1, 0, 0)
  point P0 (0, 0)
  point P1 (80.085, 10.73)
  point P2 (85.165, 10.73)
  point P3 (82.625, 10.73)
  point P4 (68.54, -8)
  point P5 (63.46, -8)
  point P6 (63.46, 8)
  point P7 (68.54, 8)
  point P8 (53.8, -28.4)
  point P9 (59.6, 27.6)
  point P10 (77.8, -26.2)
  point P11 (57.6, -36.1)
  constraints: 11 other
hole "Hole7" at (80.085, 10.73, 0.5) at (85.165, 10.73, 0.5) at (82.625, 10.73, 0.5) direction (0, 0, -1) diameter 1.6 end through all
hole "Hole8" at (68.54, -8, 0.5) at (63.46, -8, 0.5) at (63.46, 8, 0.5) at (68.54, 8, 0.5) direction (0, 0, -1) diameter 1.1 end through all
hole "Hole9" at (59.6, 27.6, 0.5) at (57.6, -36.1, 0.5) at (53.8, -28.4, 0.5) at (77.8, -26.2, 0.5) direction (0, 0, -1) diameter 1 end through all
equation "\"d23\" = d22"
equation "\"d25\" = d22"
equation "\"d12\" = d11"
body "Solid1"
